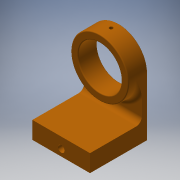
# Autodesk Inventor part: Equerre-Potar
Saved by Autodesk Inventor 2016 SP1 (Build 200210100, 210)
## iProperties
Created: 2016-01-27
Part Number: Equerre-Potar
Material: Plastique ABS
Document SubType Name: Modeling
Designer: sd
Mass: 39.859 g
Surface Area: 66.2058 cm^2
Volume: 37.6029 cm^3
Density: 1.06 g/cm^3
Appearance: Orange
Author: sd
Autodesk Inventor part; units mm, degrees
ref_plane "YZ Plane" through (0, 0, 0) normal (1, 0, 0) x (0, 1, 0)
ref_plane "XZ Plane" through (0, 0, 0) normal (0, 1, 0) x (-1, 0, 0)
sketch "Esquisse1" plane through (0, 0, 0) normal (0, 1, 0) x (-1, 0, 0)
  line L0 (-15, -15) -> (15, -15)
  line L1 (15, -15) -> (15, 15)
  line L2 (15, 15) -> (-15, 15)
  line L3 (-15, 15) -> (-15, -15)
  circle A0 centre (0, 15) radius 15
  point P0 (0, 0)
  dimension "d0" = 30
  dimension "d1" = 30
  dimension "d2" = 15
  dimension "d3" = 30
  dimension "d4" = 15
  constraints: 8 end point, 2 parallel, 1 centre point, 1 horizontal, 1 midpoint, 1 perpendicular
  measures "d0" diameter of A0
  measures "d1" distance between parallel lines of L1 L3
  measures "d2" horizontal distance of point (0, 0) L0.start
  measures "d3" distance of L0.start L2.end
  measures "d4" horizontal distance of point (0, 0) L0.start
extrude "Extrusion1" add sketch "Esquisse1" along normal blind 30
sketch "Esquisse2" plane through (0, 0, 0) normal (0, -1, 0) x (1, 0, 0)
  line L0 (15, -15) -> (-15, -15) projected
  line L1 (-16, -6) -> (16, -6)
  line L2 (16, -6) -> (16, 32)
  line L3 (16, 32) -> (-16, 32)
  line L4 (-16, 32) -> (-16, -6)
  point P0 (0, 0)
  dimension "d7" = 16
  dimension "d8" = 32
  dimension "d10" = 9
  dimension "d11" = 38
  constraints: 8 end point, 2 parallel, 1 horizontal, 1 perpendicular
  measures "d7" horizontal distance of L1.start point (0, 0)
  measures "d8" distance of L2.end L3.end
  measures "d10" distance between parallel lines of L0 L1
  measures "d11" distance between parallel lines of L1 L3
extrude "Extrusion2" cut sketch "Esquisse2" against normal blind 20
sketch "Esquisse3" plane through (0, 20, 0) normal (0, -1, 0) x (1, 0, 0)
  line L0 (-15, -6) -> (-15, 15) projected
  line L1 (15, -6) -> (-15, -6) projected
  line L2 (15, 15) -> (15, -6) projected
  arc A0 (15, 15) -> (-15, 15) centre (0, 15) ccw projected
  line L3 (-18.5, -6) -> (18.5, -6)
  line L4 (18.5, -6) -> (18.5, 32)
  line L5 (18.5, 32) -> (-18.5, 32)
  line L6 (-18.5, 32) -> (-18.5, -6)
  line L7 (15, -15) -> (-15, -15) projected
  circle A1 centre (0, 15) radius 15
  point P0 (0, 0)
  dimension "d14" = 38
  dimension "d15" = 9
  dimension "d16" = 37
  dimension "d17" = 18.5
  dimension "d18" = 30
  constraints: 8 end point, 2 parallel, 1 centre point, 1 coincident, 1 horizontal, 1 perpendicular
  measures "d14" distance of L5.end L3.start
  measures "d15" distance from line of L7 L3.start
  measures "d16" distance of L4.end L5.end
  measures "d17" horizontal distance of A0.centre L5.end
  measures "d18" diameter of A1
extrude "Extrusion3" cut sketch "Esquisse3" against normal blind 7 contours L0 A1 L2 L1
sketch "Esquisse4" plane through (0, 20, 15) normal (0, -1, 0) x (1, 0, 0)
  circle A0 centre (0, 0) radius 15 projected
  circle A1 centre (0, 0) radius 11.25
  point P0 (0, -15)
  dimension "d21" = 22.5
  constraints: 1 centre point, 1 coincident, 1 vertical alignment
  measures "d21" diameter of A1
extrude "Extrusion4" cut sketch "Esquisse4" against normal through all contours A1
fillet "Congé1" radius 3 1 edges at (0, 27, -6)
fillet "Congé2" radius 3 1 edges at (0, 27, 0)
sketch "Esquisse5" plane through (0, 30, 0) normal (0, 1, 0) x (1, 0, 0)
  line L0 (15, 15) -> (-15, 15) projected
  line L1 (3.5, 15) -> (-3.5, 15)
  line L2 (-3.5, 15) -> (-3.5, 11.5)
  line L3 (-3.5, 11.5) -> (3.5, 11.5)
  line L4 (3.5, 11.5) -> (3.5, 15)
  circle A0 centre (0, 11.5) radius 3.5
  point P0 (0, 0)
  dimension "d27" = 7
  dimension "d28" = 3.5
  dimension "d29" = 3.5
  dimension "d30" = 7
  constraints: 8 end point, 2 parallel, 1 centre point, 1 horizontal, 1 midpoint, 1 perpendicular, 1 point on line
  measures "d27" distance of L2.end L3.end
  measures "d28" horizontal distance of point (0, 0) L1.start
  measures "d29" distance of L1.start L3.end
  measures "d30" diameter of A0
extrude "Extrusion5" cut sketch "Esquisse5" against normal blind 27
sketch "Esquisse6" plane through (0, 3, 0) normal (0, 1, 0) x (1, 0, 0)
  arc A0 (-3.5, 11.5) -> (3.5, 11.5) centre (0, 11.5) ccw projected
  circle A1 centre (0, 11.5) radius 1.75
  point P0 (0, 0)
  dimension "d33" = 3.5
  constraints: 1 centre point, 1 coincident
  measures "d33" diameter of A1
extrude "Extrusion6" cut sketch "Esquisse6" against normal through all
ref_plane "Plan de construction1" through (0, 0, 30) normal (0, 0, 1) x (1, 0, 0)
sketch "Esquisse7" plane through (0, 0, 30) normal (0, 0, 1) x (1, 0, 0)
  circle A0 centre (0, 26) radius 0.9
  line L0 (15, 30) -> (-15, 30) projected
  line L1 (-15, 0) -> (-15, 30) projected
  point P0 (0, 0)
  dimension "d36" = 1.8
  dimension "d37" = 4
  dimension "d38" = 15
  constraints: 1 centre point
  measures "d36" diameter of A0
  measures "d37" distance from line of L0 A0.centre
  measures "d38" distance from line of L1 A0.centre
extrude "Extrusion7" cut sketch "Esquisse7" against normal blind 5
fillet "Congé3" radius 0.5 6 edges at (-11.25, 30, 15) (-11.25, 20, 15) (15, 20, 15) (15, 30, 0) (-15, 30, 0) (0, 30, 30)
equation "\"d1\" = d0"
equation "\"d2\" = 0.5 * d1"
equation "\"d4\" = 0.5 * d3"
equation "\"d8\" = 2 * d7"
equation "\"d17\" = 0.5 * d16"
equation "\"d28\" = 0.5 * d27"
equation "\"d29\" = d28"
equation "\"d30\" = d27"
